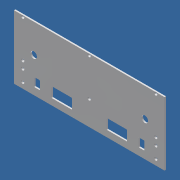
# Autodesk Inventor part: J001397
Saved by Autodesk Inventor 2012 SP2 (Build 160219200, 219)
## iProperties
Created: 2012-06-04
Part Number: J001397
Material: ALUMINUM, 6061-T651
Vendor: HHMI: JFRC - ID&F
Document SubType Name: Modeling
Designer: NEGRASHOVI
Density: 2.7 g/cm^3
Project: P-51601
Mass: 369.474 g
Surface Area: 911.514 cm^2
Volume: 136.842 cm^3
Description: FRONT PANEL
RuleStatus: InUse
AfterDocSave0: file://Part Number Cleaner
LAB/DEPT: GONEN (LAB)
REQUESTING SCIENTIST: GONEN, TAMIR
SURFACE ROUGHNESS: 32 Ra
DESIGN DEPARTMENT: HHMI: JFRC - ID&F
SPECIAL FINISH: ANODIZE PER MIL-A-8625F, TYPE II, CLASS 2 (BLACK)
ALTERED ITEM PART NUMBER: N/A
ALTERED ITEM VENDOR: N/A
ALTERED ITEM DESCRIPTION: N/A
Author: NEGRASHOVI
Revision Number: -
Autodesk Inventor part; units mm, degrees
ref_plane "YZ Plane" through (0, 0, 0) normal (1, 0, 0) x (0, 1, 0)
ref_plane "XZ Plane" through (0, 0, 0) normal (0, 1, 0) x (-1, 0, 0)
ref_plane "XY Plane" through (0, 0, 0) normal (0, 0, 1) x (1, 0, 0)
sketch "Sketch1" plane through (0, 0, 0) normal (0, 0, 1) x (1, 0, 0)
  line L0 (-165.1, 69.85) -> (165.1, 69.85)
  line L1 (165.1, 69.85) -> (165.1, -69.85)
  line L2 (165.1, -69.85) -> (-165.1, -69.85)
  line L3 (-165.1, -69.85) -> (-165.1, 69.85)
  point P0 (0, 0)
  dimension "d0" = 139.7
  dimension "d1" = 330.2
  dimension "d2" = 69.85
  dimension "d3" = 165.1
  constraints: 8 end point, 2 parallel, 1 horizontal, 1 perpendicular
  measures "d0" distance of L0.end L1.end
  measures "d1" distance of L0.start L0.end
  measures "d2" distance from line of point (0, 0) L0
  measures "d3" distance from line of L1 point (0, 0)
extrude "Extrusion1" add sketch "Sketch1" along normal blind 3.175
sketch "Sketch2" plane through (0, 0, 3.175) normal (0, 0, 1) x (1, 0, 0)
  line L0 (0, -97.79) -> (0, 97.79) construction
  line L1 (-162.2078, 6.35) -> (163.5203, 6.35) construction
  line L2 (-165.1, 69.85) -> (165.1, 69.85) projected
  point P0 (0, 0)
  point P1 (-121.92, 6.35)
  point P2 (121.92, 6.35)
  dimension "d6" = 121.92
  dimension "d23" = 63.5
  constraints: 2 end point, 1 horizontal, 1 point on line, 1 symmetric about line
  measures "d6" distance from line of point (-121.92, 6.35) L0
  measures "d23" distance between parallel lines of L1 L2
hole "Hole1" at (-121.92, 6.35, 3.175) at (121.92, 6.35, 3.175) direction (0, 0, -1) diameter 14.2875 end through all
sketch "Sketch4" plane through (0, 0, 3.175) normal (0, 0, 1) x (1, 0, 0)
  line L0 (-165.1, 69.85) -> (165.1, 69.85) projected
  line L1 (-165.1, -69.85) -> (-165.1, 69.85) projected
  line L2 (165.1, -69.85) -> (-165.1, -69.85) projected
  line L3 (165.1, 69.85) -> (165.1, -69.85) projected
  line L4 (-165.1, -15.875) -> (165.1, -15.875) construction
  line L5 (0, 69.85) -> (0, -69.85) construction
  line L6 (-146.05, 69.85) -> (-146.05, -69.85) construction
  line L7 (-165.1, 66.675) -> (165.1, 66.675) construction
  point P0 (0, 0)
  point P1 (-146.05, -15.875)
  point P2 (146.05, -15.875)
  point P3 (0, -15.875)
  point P4 (-146.05, -31.75)
  point P5 (-146.05, -57.15)
  point P6 (146.05, -31.75)
  point P7 (146.05, -57.15)
  point P8 (0, 66.675)
  point P9 (-146.05, 66.675)
  point P10 (146.05, 66.675)
  dimension "d24" = 85.725
  dimension "d49" = 12.7
  dimension "d50" = 25.4
  dimension "d51" = 3.175
  dimension "d58" = 146.05
  constraints: 15 point on line, 8 end point, 4 midpoint, 4 symmetric about line, 2 horizontal, 1 vertical
  measures "d24" distance between parallel lines of L4 L0
  measures "d49" distance from line of point (-146.05, -57.15) L2
  measures "d50" distance of point (-146.05, -31.75) point (-146.05, -57.15)
  measures "d51" distance between parallel lines of L7 L0
  measures "d58" distance between parallel lines of L5 L6
hole "Hole3" at (-146.05, -15.875, 3.175) at (146.05, -15.875, 3.175) at (0, -15.875, 3.175) at (-146.05, -31.75, 3.175) at (-146.05, -57.15, 3.175) at (146.05, -31.75, 3.175) at (146.05, -57.15, 3.175) at (-146.05, 66.675, 3.175) at (146.05, 66.675, 3.175) at (0, 66.675, 3.175) direction (0, 0, -1) diameter 3.81 end through all countersink diameter 7.0866 countersink angle 82 clearance for "Flat Head Machine Screw (82)" size "#6" standard "Ansi Unified Screw Threads"
sketch "Sketch5" plane through (0, 0, 3.175) normal (0, 0, 1) x (1, 0, 0)
  line L0 (-83.1, -33.2) -> (-38.1, -33.2)
  line L1 (-38.1, -33.2) -> (-38.1, -55.7)
  line L2 (-38.1, -55.7) -> (-83.1, -55.7)
  line L3 (-83.1, -55.7) -> (-83.1, -33.2)
  line L4 (0, -97.79) -> (0, 97.79) construction
  line L5 (165.1, -69.85) -> (-165.1, -69.85) construction
  line L6 (-155.899, -44.45) -> (168.0806, -44.45) construction
  line L7 (-121.2, -34.925) -> (-108.5, -34.925)
  line L8 (-108.5, -34.925) -> (-108.5, -53.975)
  line L9 (-108.5, -53.975) -> (-121.2, -53.975)
  line L10 (-121.2, -53.975) -> (-121.2, -34.925)
  line L11 (83.1, -33.2) -> (38.1, -33.2)
  line L12 (38.1, -33.2) -> (38.1, -55.7)
  line L13 (38.1, -55.7) -> (83.1, -55.7)
  line L14 (83.1, -55.7) -> (83.1, -33.2)
  line L15 (121.2, -34.925) -> (108.5, -34.925)
  line L16 (108.5, -34.925) -> (108.5, -53.975)
  line L17 (108.5, -53.975) -> (121.2, -53.975)
  line L18 (121.2, -53.975) -> (121.2, -34.925)
  point P0 (0, 0)
  dimension "d33" = 45
  dimension "d36" = 38.1
  dimension "d53" = 25.4
  dimension "d54" = 22.5
  dimension "d55" = 12.7
  dimension "d56" = 19.05
  dimension "d57" = 25.4
  constraints: 34 end point, 8 symmetric about line, 4 parallel, 3 horizontal, 2 perpendicular, 2 other
  measures "d33" distance of L1.end L2.end
  measures "d36" distance between parallel lines of L1 L4
  measures "d53" distance between parallel lines of L6 L5
  measures "d54" distance of L0.end L1.end
  measures "d55" distance of L7.start L7.end
  measures "d56" distance of L9.end L7.start
  measures "d57" distance between parallel lines of L8 L3
extrude "Extrusion2" cut sketch "Sketch5" against normal up to next
fillet "Fillet1" radius 1.5875 16 edges at (-121.2, -53.975, 1.5875) (-83.1, -55.7, 1.5875) (38.1, -55.7, 1.5875) (108.5, -53.975, 1.5875) (-108.5, -53.975, 1.5875) (-38.1, -55.7, 1.5875) (83.1, -55.7, 1.5875) (121.2, -53.975, 1.5875) (121.2, -34.925, 1.5875) (83.1, -33.2, 1.5875) (-38.1, -33.2, 1.5875) (-108.5, -34.925, 1.5875) (108.5, -34.925, 1.5875) (38.1, -33.2, 1.5875) (-83.1, -33.2, 1.5875) (-121.2, -34.925, 1.5875)
equation "\"d2\" = 0.5 * d0"
equation "\"d3\" = 0.5 * d1"
body "Solid1"
